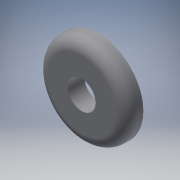
# Autodesk Inventor part: SecindaryCap
Saved by Autodesk Inventor 2019 (Build 230136000, 136)
## iProperties
Created: 2021-01-17
Part Number: SecindaryCap
Material: Типовые
Document SubType Name: Modeling
Designer: Dazer
Density: 1 g/cm^3
Appearance: По умолчанию
Author: Dazer
Autodesk Inventor part; units mm, degrees
ref_plane "YZ Plane" through (0, 0, 0) normal (1, 0, 0) x (0, 1, 0)
ref_plane "XZ Plane" through (0, 0, 0) normal (0, 1, 0) x (-1, 0, 0)
ref_plane "XY Plane" through (0, 0, 0) normal (0, 0, 1) x (1, 0, 0)
sketch "Эскиз1" plane through (0, 0, 0) normal (0, 0, 1) x (1, 0, 0)
  line L0 (-4.0768, 1.9994) -> (-0.6127, 3.9994) projected
  line L1 (-0.6127, 3.9994) -> (2.8514, 1.9994) projected
  line L2 (2.8514, 1.9994) -> (2.8353, 0.4994) projected
  line L3 (2.8353, 0.4994) -> (7.3716, 0.4994) projected
  arc A0 (7.3716, 0.4994) -> (7.3716, -0.5006) centre (-0.6127, -0.0006) ccw projected
  line L4 (7.3716, -0.5006) -> (2.8246, -0.5006) projected
  line L5 (2.8246, -0.5006) -> (2.8082, -2.0255) projected
  line L6 (2.8082, -2.0255) -> (-0.6127, -4.0006) projected
  line L7 (-0.6127, -4.0006) -> (-4.0768, -2.0006) projected
  line L8 (-4.0768, -2.0006) -> (-4.0768, 1.9994) projected
  circle A1 centre (-0.6127, -0.0006) radius 8
  point P0 (0, 0)
  constraints: 1 centre point, 1 coincident, 1 concentric
extrude "Выдавливание1" add sketch "Эскиз1" along normal blind 3
fillet "Сопряжение1" radius 2 1 edges at (-8.6127, -0.0006, 3)
sketch "Эскиз2" plane through (-0.6127, -0.0006, 3) normal (0, 0, 1) x (1, 0, 0)
  circle A0 centre (0, 0) radius 2.5
  point P0 (0.6127, 0.0006)
  dimension "d3" = 5
  constraints: 1 centre point
  measures "d3" diameter of A0
extrude "Выдавливание2" cut sketch "Эскиз2" against normal blind 3
